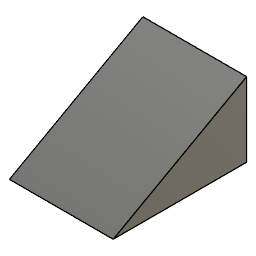
Ex1-lab1 (Autodesk Fusion 360 design; units mm, degrees)
part number: 2026-03-02-18-06-11-680
Autodesk Fusion 360 part; units mm, degrees
sketch "Sketch1" plane through (0, 0, 0) normal (0, 0, 1) x (1, 0, 0)
  line L0 (50, 50) -> (50, 25)
  line L1 (50, 25) -> (95, 25)
  line L2 (95, 25) -> (50, 50)
  dimension "d1" = 25
  dimension "d2" = 45
  constraint vertical L0
  constraint perpendicular L0 L1
  measures "d1" distance of L0.start L0.end
  measures "d2" distance of L0.end L1.end
extrude "Extrude1" add sketch "Sketch1" along normal blind 35
move_body "Move1" bodies 1 to x (0, -1, 0) y (0, 0, 1) z (-1, 0, 0) at (72.5, 110, -37.5)
move_body "Move2" bodies 1 to x (1, 0, 0) y (0, 1, 0) z (0, 0, 1) at (0, 30, 0)
